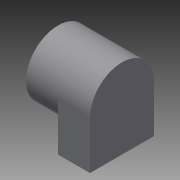
# Autodesk Inventor part: uchwytG5
Saved by Autodesk Inventor 2014 (Build 180170000, 170)
## iProperties
Created: 2013-12-25
Part Number: uchwytG5
Material: Ogólny
Document SubType Name: Modeling
Designer: Kuba
Density: 1 g/cm^3
Appearance: Domyślna
d0: 20,000 mm
d3: 15,000 mm
d4: 10,000 mm
d5: 0,00 deg
d6: 10,000 mm
d7: 0,00 deg
d8: 16,000 mm
d9: 2,000 mm
d10: 2,000 ul
d12: 8,000 mm
d17: 10,000 mm
d18: 0,00 deg
d19: 17,000 mm
d20: 0,00 deg
Author: Kuba
Autodesk Inventor part; units mm, degrees
ref_plane "YZ Plane" through (0, 0, 0) normal (1, 0, 0) x (0, 1, 0)
ref_plane "XZ Plane" through (0, 0, 0) normal (0, 1, 0) x (-1, 0, 0)
ref_plane "XY Plane" through (0, 0, 0) normal (0, 0, 1) x (1, 0, 0)
sketch "Szkic1" plane through (0, 0, 0) normal (1, 0, 0) x (0, 1, 0)
  circle A0 centre (0, 0) radius 10
  line L0 (-14, 0) -> (14, 0) projected
  line L1 (0, -20) -> (0, 15) projected
  line L2 (10, 0) -> (10, -15)
  line L3 (-10, -15) -> (10, -15)
  line L4 (-10, 0) -> (-10, -15)
  dimension "d0" = 20
  dimension "d3" = 15
  constraints: 6 end point, 2 parallel, 2 point on line, 2 tangent, 1 centre point, 1 coincident, 1 perpendicular
  measures "d0" diameter of A0
  measures "d3" distance of L2.start L2.end
extrude "Wyciągnięcie proste2" add sketch "Szkic1" along normal blind 10
extrude "Wyciągnięcie proste3" add sketch "Szkic1" against normal blind 10 contours L0 L1 A0 | A0 L1 L0 | L1 L0 A0 | A0 L0 L1
sketch "Szkic2" plane through (-10, 0, 0) normal (-1, 0, 0) x (0, 0, 1)
  circle A0 centre (0, 0) radius 10 projected
  circle A1 centre (0, 0) radius 8
  line L0 (-20, 0) -> (15, 0) projected
  line L1 (0, -14) -> (0, 14) projected
  circle A2 centre (-4, 0) radius 1
  circle A3 centre (4, 0) radius 1
  dimension "d8" = 16
  dimension "d9" = 2
  dimension "d12" = 8
  constraints: 3 centre point, 1 coincident, 1 horizontal, 3 other
  measures "d8" diameter of A1
  measures "d9" diameter of A2
  measures "d12" distance of A2.centre A3.centre
extrude "Wyciągnięcie proste4" cut sketch "Szkic2" against normal blind 10 contours L0 A3 L1 A1 | A1 L1 L0 A3 | L1 L0 A2 A1 | A1 L0 A2 L1
extrude "Wyciągnięcie proste5" cut sketch "Szkic2" against normal blind 17 contours A3 L0 | L0 A3 | A2 L0 | L0 A2
equation "\"d12\" = 0.5 * d8"
